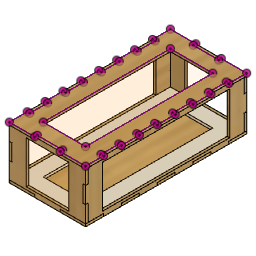
probatio-base-parametric-generator (Autodesk Fusion 360 design; units mm, degrees)
Autodesk Fusion 360 part; units mm, degrees
note: some values were not read from the file. Set by a fixed rule: which sketch regions a step uses.
sketch "Bottom Panel Profile Sketch" plane through (0, 0, 0) normal (0, 0, 1) x (1, 0, 0) in component "Main Box"
  line L0 (0, 0) -> (90, 0)
  line L1 (90, 0) -> (90, 190)
  line L2 (90, 190) -> (0, 190)
  line L3 (0, 190) -> (0, 0)
  dimension "d21" = 90
  dimension "d22" = 190
  constraint horizontal L0
  constraint vertical L1
  constraint horizontal L2
  constraint vertical L3
  constraint coincident L0.start L3.end
  measures "d21" distance of L0.start L0.end
  measures "d22" distance of L0.start L2.end
extrude "Bottom Panel Extrude" add sketch "Bottom Panel Profile Sketch" along normal blind 3 makes body 1 in component "Main Box"
sketch "Bottom Panel Front Fingers Sketch" plane through (0, 0, 0) normal (0, -1, 0) x (1, 0, 0) in component "Main Box"
  line L0 (0, 0) -> (90, 0)
  line L1 (90, 0) -> (90, 3)
  line L2 (90, 3) -> (0, 3)
  line L3 (0, 3) -> (0, 0)
  line L4 (45, 3) -> (45, 0) construction
  line L5 (30, 1.5) -> (60, 1.5) construction
  line L6 (30, 0) -> (60, 0)
  line L7 (60, 0) -> (60, 3)
  line L8 (60, 3) -> (30, 3)
  line L9 (30, 3) -> (30, 0)
  dimension "d25" = 30
  dimension "d26" = 30
  constraint midpoint L2 L4.start
  constraint midpoint L0 L4.end
  constraint perpendicular L4 L5
  constraint midpoint L4 L5
  constraint horizontal L6
  constraint vertical L7
  constraint horizontal L8
  constraint vertical L9
  constraint coincident L2 L7.end
  constraint coincident L0 L6.start
  constraint coincident L5.start L9
  measures "d25" horizontal distance of L7.end L8.end
  measures "d26" horizontal distance of L5.start L5.end
extrude "Bottom Panel Front Finger Extrude" cut sketch "Bottom Panel Front Fingers Sketch" against normal blind 3 contours L0 L2 L6 L7 L8 L9 bodies 1 in component "Main Box"
pattern_linear "Bottom Panel Length Fingers Pattern" count 1 spacing 0 along (1, 0, 0) count 2 spacing 187 along (0, 1, 0) of "Bottom Panel Front Finger Extrude" in component "Main Box"
sketch "Bottom Panel Left Fingers Sketch" plane through (0, 0, 0) normal (-1, 0, 0) x (0, -1, 0) in component "Main Box"
  line L0 (-190, 0) -> (0, 0)
  line L1 (0, 0) -> (0, 3)
  line L2 (0, 3) -> (-190, 3)
  line L3 (-190, 3) -> (-190, 0)
  line L4 (-95, 3) -> (-95, 0) construction
  line L5 (-168.8889, 1.5) -> (-21.1111, 1.5) construction
  line L6 (-21.1111, 0) -> (-42.2222, 0)
  line L7 (-42.2222, 0) -> (-42.2222, 3)
  line L8 (-42.2222, 3) -> (-21.1111, 3)
  line L9 (-21.1111, 3) -> (-21.1111, 0)
  dimension "d33" = 21.1111
  dimension "d34" = 147.7778
  constraint midpoint L2 L4.start
  constraint midpoint L0 L4.end
  constraint perpendicular L4 L5
  constraint midpoint L4 L5
  constraint horizontal L6
  constraint vertical L7
  constraint horizontal L8
  constraint vertical L9
  constraint coincident L2 L7.end
  constraint coincident L0 L6.start
  constraint coincident L5.end L9
  measures "d33" horizontal distance of L6.start L6.end
  measures "d34" horizontal distance of L5.start L5.end
extrude "Bottom Panel Left Finger Extrude" cut sketch "Bottom Panel Left Fingers Sketch" against normal blind 3 contours L0 L2 L6 L7 L8 L9 bodies 1 in component "Main Box"
pattern_linear "Bottom Panel Width Fingers Pattern" count 4 spacing 42.2222 along (0, 1, 0) count 2 spacing 87 along (1, 0, 0) of "Bottom Panel Left Finger Extrude" in component "Main Box"
sketch "Front Panel Profile Sketch" plane through (0, 0, 0) normal (0, 1, 0) x (1, 0, 0) in component "Main Box"
  line L0 (0, 0) -> (90, 0)
  line L1 (90, 0) -> (90, -62)
  line L2 (90, -62) -> (0, -62)
  line L3 (0, -62) -> (0, 0)
  dimension "d41" = 90
  dimension "d42" = 62
  constraint horizontal L0
  constraint vertical L1
  constraint horizontal L2
  constraint vertical L3
  constraint coincident L0.start L3.end
  measures "d41" distance of L0.start L0.end
  measures "d42" distance of L0.start L2.end
extrude "Front Panel Extrude" add sketch "Front Panel Profile Sketch" along normal blind 3 separate body makes body 2 in component "Main Box"
combine "Front Panel Combine" operation cut target body 2 tool bodies 1 keep tools in component "Main Box"
sketch "Front Panel Left Fingers Sketch" plane through (0, 0, 0) normal (0, -1, 0) x (1, 0, 0) in component "Main Box"
  line L0 (90, 3) -> (90, 62)
  line L1 (90, 62) -> (0, 62)
  line L2 (0, 62) -> (0, 3)
  line L3 (0, 3) -> (30, 3)
  line L4 (30, 3) -> (30, 0)
  line L5 (30, 0) -> (60, 0)
  line L6 (60, 0) -> (60, 3)
  line L7 (60, 3) -> (90, 3)
  line L8 (0, 32.5) -> (3, 32.5) construction
  line L9 (1.5, 42.3333) -> (1.5, 22.6667) construction
  line L10 (0, 22.6667) -> (3, 22.6667)
  line L11 (3, 22.6667) -> (3, 42.3333)
  line L12 (3, 42.3333) -> (0, 42.3333)
  line L13 (0, 42.3333) -> (0, 22.6667)
  dimension "d45" = 3
  dimension "d46" = 19.6667
  dimension "d47" = 19.6667
  constraint midpoint L2 L8.start
  constraint perpendicular L2 L8
  constraint perpendicular L8 L9
  constraint midpoint L8 L9
  constraint horizontal L10
  constraint vertical L11
  constraint horizontal L12
  constraint vertical L13
  constraint coincident L2 L10.start
  constraint coincident L9.end L10
  constraint coincident L8.end L11
  measures "d45" distance of L8.start L8.end
  measures "d46" vertical distance of L10.start L12.end
  measures "d47" vertical distance of L9.start L9.end
extrude "Front Panel Left Fingers Extrude" cut sketch "Front Panel Left Fingers Sketch" against normal blind 3 contours L2 L10 L11 L12 L13 bodies 2 in component "Main Box"
pattern_linear "Front Panel Height Fingers Pattern" count 1 spacing 0 along (0, 0, 1) count 2 spacing 87 along (1, 0, 0) of "Front Panel Left Fingers Extrude" in component "Main Box"
pattern_linear "Front Panel Pattern" count 2 spacing 187 along (0, 1, 0) of bodies 2 makes body 3 in component "Main Box"
sketch "Left Panel Profile Sketch" plane through (0, 0, 0) normal (1, 0, 0) x (0, 1, 0) in component "Main Box"
  line L0 (0, 0) -> (190, 0)
  line L1 (190, 0) -> (190, 62)
  line L2 (190, 62) -> (0, 62)
  line L3 (0, 62) -> (0, 0)
  dimension "d58" = 190
  dimension "d59" = 62
  constraint horizontal L0
  constraint vertical L1
  constraint horizontal L2
  constraint vertical L3
  constraint coincident L0.start L3.end
  measures "d58" distance of L0.start L0.end
  measures "d59" distance of L0.start L2.end
extrude "Left Panel Extrude" add sketch "Left Panel Profile Sketch" along normal blind 3 separate body makes body 4 in component "Main Box"
sketch "Left Panel Front Fingers Sketch" plane through (0, 0, 0) normal (0, -1, 0) x (1, 0, 0) in component "Main Box"
  line L0 (0, 62) -> (0, 0)
  line L1 (0, 0) -> (3, 0)
  line L2 (3, 0) -> (3, 62)
  line L3 (3, 62) -> (0, 62)
  line L4 (0, 62) -> (3, 62)
  line L5 (3, 62) -> (3, 42.3333)
  line L6 (3, 42.3333) -> (0, 42.3333)
  line L7 (0, 42.3333) -> (0, 62)
  dimension "d72" = 19.6667
  constraint horizontal L4
  constraint vertical L5
  constraint horizontal L6
  constraint vertical L7
  constraint coincident L2 L5.end
  constraint coincident L0.start L3.end
  measures "d72" vertical distance of L0.start L6.end
extrude "Left Panel Front Fingers Extrude" cut sketch "Left Panel Front Fingers Sketch" against normal blind 3 contours L0 L2 L3 L4 L5 L6 L7 bodies 4 in component "Main Box"
pattern_linear "Left Panel Slots Pattern" count 2 spacing 187 along (0, 1, 0) of "Left Panel Front Fingers Extrude" in component "Main Box"
combine "Left Panel Combine" operation cut target body 4 tool bodies 3 1 2 keep tools in component "Main Box"
extrude "Extrude11" add 1 faces at (0, 91.4815, 42.3333) along direction (-1, 0, 0) blind 3 from surface at -90 separate body on bodies 4 makes body 5 in component "Main Box"
extrude "Extrude9" cut 1 faces at (50, 29.1481, 3) along direction (0, 0, -1) blind 3 from surface at -59 on bodies 1 bodies 2 3 4 5 in component "Main Box"
extrude "Extrude12" add 1 faces at (50, 29.1481, 0) along direction (0, 0, -1) blind 3 from surface at -62 separate body on bodies 1 makes body 6 in component "Main Box"
sketch "Sketch8" plane through (0, 190, 0) normal (0, 1, 0) x (-1, 0, 0) in component "Main Box"
  line L0 (-90, 59) -> (-90, 42.3333)
  line L1 (-90, 42.3333) -> (-87, 42.3333)
  line L2 (-87, 42.3333) -> (-87, 22.6667)
  line L3 (-87, 22.6667) -> (-90, 22.6667)
  line L4 (-90, 22.6667) -> (-90, 3)
  line L5 (-90, 3) -> (-60, 3)
  line L6 (-60, 3) -> (-60, 0)
  line L7 (-60, 0) -> (-30, 0)
  line L8 (-30, 0) -> (-30, 3)
  line L9 (-30, 3) -> (0, 3)
  line L10 (0, 3) -> (0, 22.6667)
  line L11 (0, 22.6667) -> (-3, 22.6667)
  line L12 (-3, 22.6667) -> (-3, 42.3333)
  line L13 (-3, 42.3333) -> (0, 42.3333)
  line L14 (0, 42.3333) -> (0, 59)
  line L15 (-30, 62) -> (-60, 62)
  line L16 (-90, 59) -> (0, 3) construction
  line L17 (0, 59) -> (-90, 3) construction
  line L18 (-20, 56) -> (-70, 56)
  line L19 (-70, 56) -> (-70, 6)
  line L20 (-70, 6) -> (-20, 6)
  line L21 (-20, 6) -> (-20, 56)
  line L22 (-20, 56) -> (-70, 6) construction
  line L23 (-70, 56) -> (-20, 6) construction
  line L24 (0, 59) -> (-30, 59)
  line L25 (-30, 59) -> (-30, 62)
  line L26 (-60, 62) -> (-60, 59)
  line L27 (-60, 59) -> (-90, 59)
  point P0 (-45, 31)
  dimension "d118" = 50
  dimension "d119" = 50
  constraint coincident L0.start L16.start
  constraint coincident L9.end L10.start
  constraint coincident L14.end L17.start
  constraint coincident L4.end L5.start
  constraint perpendicular L18 L19
  constraint parallel L18 L20
  constraint parallel L19 L21
  constraint horizontal L18
  constraint coincident L22 P0
  constraint coincident L23 P0
  constraint midpoint L16 P0
  measures "d118" distance of L18.end L19.end
  measures "d119" distance of L19.end L20.end
extrude "Extrude10" cut sketch "Sketch8" against normal blind 3 contours L18 L19 L20 L21 bodies 3 in component "Main Box"
sketch "Sketch9" plane through (0, 0, 62) normal (0, 0, 1) x (-1, 0, 0) in component "Main Box"
  line L0 (-90, -190) -> (-60, -190)
  line L1 (-60, -190) -> (-60, -187)
  line L2 (-60, -187) -> (-30, -187)
  line L3 (-30, -187) -> (-30, -190)
  line L4 (-30, -190) -> (0, -190)
  line L5 (0, -63.3333) -> (0, -42.2222)
  line L6 (0, -42.2222) -> (-3, -42.2222)
  line L7 (-3, -42.2222) -> (-3, -21.1111)
  line L8 (-3, -21.1111) -> (0, -21.1111)
  line L9 (0, -21.1111) -> (0, 0)
  line L10 (0, 0) -> (-30, 0)
  line L11 (-30, 0) -> (-30, -3)
  line L12 (-30, -3) -> (-60, -3)
  line L13 (-60, -3) -> (-60, 0)
  line L14 (-60, 0) -> (-90, 0)
  line L15 (-90, 0) -> (-90, -21.1111)
  line L16 (-90, -21.1111) -> (-87, -21.1111)
  line L17 (-87, -21.1111) -> (-87, -42.2222)
  line L18 (-87, -42.2222) -> (-90, -42.2222)
  line L19 (-90, -42.2222) -> (-90, -63.3333)
  line L20 (-90, -147.7778) -> (-87, -147.7778)
  line L21 (-87, -147.7778) -> (-87, -168.8889)
  line L22 (-87, -168.8889) -> (-90, -168.8889)
  line L23 (-90, -168.8889) -> (-90, -190)
  line L24 (0, -190) -> (0, -168.8889)
  line L25 (0, -168.8889) -> (-3, -168.8889)
  line L26 (-3, -168.8889) -> (-3, -147.7778)
  line L27 (-3, -147.7778) -> (0, -147.7778)
  line L28 (0, -147.7778) -> (0, -126.6667)
  line L29 (0, -126.6667) -> (-3, -126.6667)
  line L30 (-3, -126.6667) -> (-3, -105.5556)
  line L31 (-3, -105.5556) -> (0, -105.5556)
  line L32 (0, -105.5556) -> (0, -84.4444)
  line L33 (0, -84.4444) -> (-3, -84.4444)
  line L34 (-3, -84.4444) -> (-3, -63.3333)
  line L35 (-3, -63.3333) -> (0, -63.3333)
  line L36 (-90, -63.3333) -> (-87, -63.3333)
  line L37 (-87, -63.3333) -> (-87, -84.4444)
  line L38 (-87, -84.4444) -> (-90, -84.4444)
  line L39 (-90, -84.4444) -> (-90, -105.5556)
  line L40 (-90, -105.5556) -> (-87, -105.5556)
  line L41 (-87, -105.5556) -> (-87, -126.6667)
  line L42 (-87, -126.6667) -> (-90, -126.6667)
  line L43 (-90, -126.6667) -> (-90, -147.7778)
  line L44 (0, -190) -> (-90, 0) construction
  line L45 (-70, -20) -> (-20, -20)
  line L46 (-20, -20) -> (-20, -170)
  line L47 (-20, -170) -> (-70, -170)
  line L48 (-70, -170) -> (-70, -20)
  line L49 (-70, -20) -> (-20, -170) construction
  line L50 (-20, -20) -> (-70, -170) construction
  point P0 (-45, -95)
  dimension "d152" = 50
  dimension "d153" = 150
  constraint coincident L4.end L24.start
  constraint coincident L14.end L15.start
  constraint perpendicular L45 L46
  constraint parallel L45 L47
  constraint parallel L46 L48
  constraint horizontal L45
  constraint coincident L49 P0
  constraint coincident L50 P0
  constraint midpoint L44 P0
  measures "d152" distance of L46.end L47.end
  measures "d153" distance of L45.end L46.end
extrude "Extrude13" cut sketch "Sketch9" against normal blind 3 contours L45 L46 L47 L48 bodies 6 in component "Main Box"
sketch "Sketch10" plane through (0, 0, 0) normal (0, -1, 0) x (1, 0, 0) in component "Main Box"
  line L0 (30, 59) -> (0, 59)
  line L1 (0, 59) -> (0, 42.3333)
  line L2 (0, 42.3333) -> (3, 42.3333)
  line L3 (3, 42.3333) -> (3, 22.6667)
  line L4 (3, 22.6667) -> (0, 22.6667)
  line L5 (0, 22.6667) -> (0, 3)
  line L6 (0, 3) -> (30, 3)
  line L7 (30, 3) -> (30, 0)
  line L8 (30, 0) -> (60, 0)
  line L9 (60, 0) -> (60, 3)
  line L10 (60, 3) -> (90, 3)
  line L11 (90, 3) -> (90, 22.6667)
  line L12 (90, 22.6667) -> (87, 22.6667)
  line L13 (87, 22.6667) -> (87, 42.3333)
  line L14 (87, 42.3333) -> (90, 42.3333)
  line L15 (90, 42.3333) -> (90, 59)
  line L16 (90, 59) -> (60, 59)
  line L17 (60, 59) -> (60, 62)
  line L18 (60, 62) -> (30, 62)
  line L19 (30, 62) -> (30, 59)
  line L20 (90, 59) -> (0, 3) construction
  line L21 (70, 6) -> (20, 6)
  line L22 (20, 6) -> (20, 56)
  line L23 (20, 56) -> (70, 56)
  line L24 (70, 56) -> (70, 6)
  line L25 (70, 6) -> (20, 56) construction
  line L26 (20, 6) -> (70, 56) construction
  point P0 (45, 31)
  dimension "d150" = 50
  dimension "d151" = 50
  constraint coincident L15.end L16.start
  constraint coincident L5.end L6.start
  constraint perpendicular L21 L22
  constraint parallel L21 L23
  constraint parallel L22 L24
  constraint horizontal L21
  constraint coincident L25 P0
  constraint coincident L26 P0
  constraint midpoint L20 P0
  measures "d150" distance of L22.end L23.end
  measures "d151" distance of L21.end L22.end
extrude "Extrude14" cut sketch "Sketch10" against normal blind 3 contours L21 L22 L23 L24 bodies 2 in component "Main Box"
sketch "Sketch11" plane through (90, 0, 0) normal (1, 0, 0) x (0, 1, 0) in component "Main Box"
  line L0 (187, 59) -> (168.8889, 59)
  line L1 (42.2222, 59) -> (42.2222, 62)
  line L2 (42.2222, 62) -> (21.1111, 62)
  line L3 (21.1111, 62) -> (21.1111, 59)
  line L4 (21.1111, 59) -> (3, 59)
  line L5 (3, 59) -> (3, 42.3333)
  line L6 (3, 42.3333) -> (0, 42.3333)
  line L7 (0, 42.3333) -> (0, 22.6667)
  line L8 (0, 22.6667) -> (3, 22.6667)
  line L9 (3, 22.6667) -> (3, 3)
  line L10 (3, 3) -> (21.1111, 3)
  line L11 (21.1111, 3) -> (21.1111, 0)
  line L12 (21.1111, 0) -> (42.2222, 0)
  line L13 (42.2222, 0) -> (42.2222, 3)
  line L14 (126.6667, 3) -> (147.7778, 3)
  line L15 (187, 3) -> (187, 22.6667)
  line L16 (187, 22.6667) -> (190, 22.6667)
  line L17 (190, 22.6667) -> (190, 42.3333)
  line L18 (190, 42.3333) -> (187, 42.3333)
  line L19 (187, 42.3333) -> (187, 59)
  line L20 (3, 59) -> (147.7778, 3) construction
  line L21 (187, 59) -> (3, 3) construction
  line L22 (170, 56) -> (20, 56)
  line L23 (20, 56) -> (20, 6)
  line L24 (20, 6) -> (170, 6)
  line L25 (170, 6) -> (170, 56)
  line L26 (170, 56) -> (20, 6) construction
  line L27 (20, 56) -> (170, 6) construction
  line L28 (168.8889, 59) -> (168.8889, 62)
  line L29 (147.7778, 62) -> (147.7778, 59)
  line L30 (147.7778, 59) -> (126.6667, 59)
  line L31 (126.6667, 59) -> (126.6667, 62)
  line L32 (126.6667, 62) -> (105.5556, 62)
  line L33 (105.5556, 62) -> (105.5556, 59)
  line L34 (105.5556, 59) -> (84.4444, 59)
  line L35 (84.4444, 59) -> (84.4444, 62)
  line L36 (84.4444, 62) -> (63.3333, 62)
  line L37 (63.3333, 62) -> (63.3333, 59)
  line L38 (63.3333, 59) -> (42.2222, 59)
  line L39 (42.2222, 3) -> (63.3333, 3)
  line L40 (63.3333, 3) -> (63.3333, 0)
  line L41 (63.3333, 0) -> (84.4444, 0)
  line L42 (84.4444, 0) -> (84.4444, 3)
  line L43 (84.4444, 3) -> (105.5556, 3)
  line L44 (105.5556, 3) -> (105.5556, 0)
  line L45 (105.5556, 0) -> (126.6667, 0)
  line L46 (126.6667, 0) -> (126.6667, 3)
  line L47 (147.7778, 3) -> (147.7778, 0)
  line L48 (147.7778, 0) -> (168.8889, 0)
  line L49 (168.8889, 0) -> (168.8889, 3)
  line L50 (168.8889, 62) -> (147.7778, 62)
  line L51 (168.8889, 3) -> (187, 3)
  point P0 (95, 31)
  dimension "d136" = 150
  dimension "d137" = 50
  constraint coincident L4.end L5.start
  constraint coincident L14.end L20.end
  constraint coincident L0.start L19.end
  constraint coincident L9.end L10.start
  constraint perpendicular L22 L23
  constraint parallel L22 L24
  constraint parallel L23 L25
  constraint horizontal L22
  constraint coincident L26 P0
  constraint coincident L27 P0
  constraint midpoint L21 P0
  measures "d136" distance of L23.end L24.end
  measures "d137" distance of L22.end L23.end
extrude "Extrude15" cut sketch "Sketch11" against normal blind 3 contours L22 L23 L24 L25 bodies 5 in component "Main Box"
sketch "Sketch12" plane through (0, 0, 0) normal (-1, 0, 0) x (0, -1, 0) in component "Main Box"
  line L0 (-187, 59) -> (-187, 42.3333)
  line L1 (-187, 42.3333) -> (-190, 42.3333)
  line L2 (-190, 42.3333) -> (-190, 22.6667)
  line L3 (-190, 22.6667) -> (-187, 22.6667)
  line L4 (-187, 22.6667) -> (-187, 3)
  line L5 (-187, 3) -> (-168.8889, 3)
  line L6 (-42.2222, 3) -> (-42.2222, 0)
  line L7 (-42.2222, 0) -> (-21.1111, 0)
  line L8 (-21.1111, 0) -> (-21.1111, 3)
  line L9 (-21.1111, 3) -> (-3, 3)
  line L10 (-3, 3) -> (-3, 22.6667)
  line L11 (-3, 22.6667) -> (0, 22.6667)
  line L12 (0, 22.6667) -> (0, 42.3333)
  line L13 (0, 42.3333) -> (-3, 42.3333)
  line L14 (-3, 42.3333) -> (-3, 59)
  line L15 (-21.1111, 59) -> (-21.1111, 62)
  line L16 (-21.1111, 62) -> (-42.2222, 62)
  line L17 (-42.2222, 62) -> (-42.2222, 59)
  line L18 (-42.2222, 59) -> (-63.3333, 59)
  line L19 (-187, 59) -> (-3, 3) construction
  line L20 (-136.5807, 56.5348) -> (-187, 3) construction
  line L21 (-20, 56) -> (-170, 56)
  line L22 (-170, 56) -> (-170, 6)
  line L23 (-170, 6) -> (-20, 6)
  line L24 (-20, 6) -> (-20, 56)
  line L25 (-20, 56) -> (-170, 6) construction
  line L26 (-170, 56) -> (-20, 6) construction
  line L27 (-3, 59) -> (-21.1111, 59)
  line L28 (-168.8889, 3) -> (-168.8889, 0)
  line L29 (-147.7778, 0) -> (-147.7778, 3)
  line L30 (-147.7778, 3) -> (-126.6667, 3)
  line L31 (-126.6667, 3) -> (-126.6667, 0)
  line L32 (-126.6667, 0) -> (-105.5556, 0)
  line L33 (-105.5556, 0) -> (-105.5556, 3)
  line L34 (-105.5556, 3) -> (-84.4444, 3)
  line L35 (-84.4444, 3) -> (-84.4444, 0)
  line L36 (-84.4444, 0) -> (-63.3333, 0)
  line L37 (-63.3333, 0) -> (-63.3333, 3)
  line L38 (-63.3333, 3) -> (-42.2222, 3)
  line L39 (-63.3333, 59) -> (-63.3333, 62)
  line L40 (-63.3333, 62) -> (-84.4444, 62)
  line L41 (-84.4444, 62) -> (-84.4444, 59)
  line L42 (-84.4444, 59) -> (-105.5556, 59)
  line L43 (-105.5556, 59) -> (-105.5556, 62)
  line L44 (-105.5556, 62) -> (-126.6667, 62)
  line L45 (-126.6667, 62) -> (-126.6667, 59)
  line L46 (-126.6667, 59) -> (-147.7778, 59)
  line L47 (-147.7778, 59) -> (-147.7778, 62)
  line L48 (-147.7778, 62) -> (-168.8889, 62)
  line L49 (-168.8889, 62) -> (-168.8889, 59)
  line L50 (-168.8889, 0) -> (-147.7778, 0)
  line L51 (-168.8889, 59) -> (-187, 59)
  point P0 (-95, 31)
  dimension "d140" = 150
  dimension "d141" = 50
  constraint coincident L0.start L19.start
  constraint coincident L9.end L10.start
  constraint coincident L4.end L5.start
  constraint perpendicular L21 L22
  constraint parallel L21 L23
  constraint parallel L22 L24
  constraint horizontal L21
  constraint coincident L25 P0
  constraint coincident L26 P0
  constraint midpoint L19 P0
  measures "d140" distance of L22.end L23.end
  measures "d141" distance of L21.end L22.end
extrude "Extrude16" cut sketch "Sketch12" against normal blind 3 contours L21 L22 L23 L24 bodies 4 in component "Main Box"
sketch "Sketch13" plane through (0, 0, 3) normal (0, 0, 1) x (-1, 0, 0) in component "Main Box"
  line L0 (-90, -190) -> (-60, -190)
  line L1 (-60, -190) -> (-60, -187)
  line L2 (-60, -187) -> (-30, -187)
  line L3 (-30, -187) -> (-30, -190)
  line L4 (-30, -190) -> (0, -190)
  line L5 (0, -190) -> (0, -168.8889)
  line L6 (0, -42.2222) -> (-3, -42.2222)
  line L7 (-3, -42.2222) -> (-3, -21.1111)
  line L8 (-3, -21.1111) -> (0, -21.1111)
  line L9 (0, -21.1111) -> (0, 0)
  line L10 (0, 0) -> (-30, 0)
  line L11 (-30, 0) -> (-30, -3)
  line L12 (-30, -3) -> (-60, -3)
  line L13 (-60, -3) -> (-60, 0)
  line L14 (-60, 0) -> (-90, 0)
  line L15 (-90, 0) -> (-90, -21.1111)
  line L16 (-90, -21.1111) -> (-87, -21.1111)
  line L17 (-87, -21.1111) -> (-87, -42.2222)
  line L18 (-87, -42.2222) -> (-90, -42.2222)
  line L19 (-90, -42.2222) -> (-90, -63.3333)
  line L20 (0, -190) -> (-90, 0) construction
  line L21 (-90, -190) -> (0, 0) construction
  line L22 (-87, -3) -> (-3, -3)
  line L23 (-3, -3) -> (-3, -187)
  line L24 (-3, -187) -> (-87, -187)
  line L25 (-87, -187) -> (-87, -3)
  line L26 (-87, -3) -> (-3, -187) construction
  line L27 (-3, -3) -> (-87, -187) construction
  line L28 (-70, -20) -> (-20, -20)
  line L29 (-20, -20) -> (-20, -170)
  line L30 (-20, -170) -> (-70, -170)
  line L31 (-70, -170) -> (-70, -20)
  line L32 (-70, -20) -> (-20, -170) construction
  line L33 (-20, -20) -> (-70, -170) construction
  line L34 (-90, -147.7778) -> (-87, -147.7778)
  line L35 (-87, -147.7778) -> (-87, -168.8889)
  line L36 (-87, -168.8889) -> (-90, -168.8889)
  line L37 (0, -168.8889) -> (-3, -168.8889)
  line L38 (-3, -168.8889) -> (-3, -147.7778)
  line L39 (-3, -147.7778) -> (0, -147.7778)
  line L40 (0, -147.7778) -> (0, -126.6667)
  line L41 (0, -126.6667) -> (-3, -126.6667)
  line L42 (-3, -126.6667) -> (-3, -105.5556)
  line L43 (-3, -105.5556) -> (0, -105.5556)
  line L44 (0, -105.5556) -> (0, -84.4444)
  line L45 (0, -84.4444) -> (-3, -84.4444)
  line L46 (-3, -84.4444) -> (-3, -63.3333)
  line L47 (-3, -63.3333) -> (0, -63.3333)
  line L48 (0, -63.3333) -> (0, -42.2222)
  line L49 (-90, -63.3333) -> (-87, -63.3333)
  line L50 (-87, -63.3333) -> (-87, -84.4444)
  line L51 (-87, -84.4444) -> (-90, -84.4444)
  line L52 (-90, -84.4444) -> (-90, -105.5556)
  line L53 (-90, -105.5556) -> (-87, -105.5556)
  line L54 (-87, -105.5556) -> (-87, -126.6667)
  line L55 (-87, -126.6667) -> (-90, -126.6667)
  line L56 (-90, -126.6667) -> (-90, -147.7778)
  line L57 (-90, -168.8889) -> (-90, -190)
  point P0 (-45, -95)
  point P1 (-45, -95)
  dimension "d144" = 84
  dimension "d145" = 184
  dimension "d146" = 50
  dimension "d147" = 150
  constraint coincident L4.end L5.start
  constraint coincident L14.end L15.start
  constraint coincident L0.start L21.start
  constraint coincident L9.end L10.start
  constraint perpendicular L22 L23
  constraint parallel L22 L24
  constraint parallel L23 L25
  constraint horizontal L22
  constraint coincident L26 P1
  constraint coincident L27 P1
  constraint midpoint L21 P1
  constraint perpendicular L28 L29
  constraint parallel L28 L30
  constraint parallel L29 L31
  constraint horizontal L28
  constraint coincident L32 P1
  constraint coincident L33 P1
  constraint coincident P1 P0
  measures "d144" distance of L23.end L24.end
  measures "d145" distance of L22.end L23.end
  measures "d146" distance of L29.end L30.end
  measures "d147" distance of L28.end L29.end
extrude "Extrude17" add sketch "Sketch13" along normal blind 3 separate body contours L2 L7 L12 L17 L22 L23 L24 L25 L35 L38 L42 L46 L50 L54 makes body 7 in component "Main Box"
sketch "Top Profile" plane through (0, 0, 62) normal (0, 0, 1) x (-1, 0, 0)
  line L0 (-20, -20) -> (-20, -170)
  line L1 (-20, -170) -> (-70, -170)
  line L2 (-70, -170) -> (-70, -20)
  line L3 (-70, -20) -> (-20, -20)
  line L4 (-90, -147.7778) -> (-87, -147.7778)
  line L5 (-87, -147.7778) -> (-87, -168.8889)
  line L6 (-87, -168.8889) -> (-90, -168.8889)
  line L7 (-90, -168.8889) -> (-90, -190)
  line L8 (-90, -190) -> (-60, -190)
  line L9 (-60, -190) -> (-60, -187)
  line L10 (-60, -187) -> (-30, -187)
  line L11 (-30, -187) -> (-30, -190)
  line L12 (-30, -190) -> (0, -190)
  line L13 (0, -190) -> (0, -168.8889)
  line L14 (0, -168.8889) -> (-3, -168.8889)
  line L15 (-3, -168.8889) -> (-3, -147.7778)
  line L16 (-3, -147.7778) -> (0, -147.7778)
  line L17 (0, -147.7778) -> (0, -126.6667)
  line L18 (0, -126.6667) -> (-3, -126.6667)
  line L19 (-3, -126.6667) -> (-3, -105.5556)
  line L20 (-3, -105.5556) -> (0, -105.5556)
  line L21 (0, -105.5556) -> (0, -84.4444)
  line L22 (0, -84.4444) -> (-3, -84.4444)
  line L23 (-3, -84.4444) -> (-3, -63.3333)
  line L24 (-3, -63.3333) -> (0, -63.3333)
  line L25 (0, -63.3333) -> (0, -42.2222)
  line L26 (0, -42.2222) -> (-3, -42.2222)
  line L27 (-3, -42.2222) -> (-3, -21.1111)
  line L28 (-3, -21.1111) -> (0, -21.1111)
  line L29 (0, -21.1111) -> (0, 0)
  line L30 (0, 0) -> (-30, 0)
  line L31 (-30, 0) -> (-30, -3)
  line L32 (-30, -3) -> (-60, -3)
  line L33 (-60, -3) -> (-60, 0)
  line L34 (-60, 0) -> (-90, 0)
  line L35 (-90, 0) -> (-90, -21.1111)
  line L36 (-90, -21.1111) -> (-87, -21.1111)
  line L37 (-87, -21.1111) -> (-87, -42.2222)
  line L38 (-87, -42.2222) -> (-90, -42.2222)
  line L39 (-90, -42.2222) -> (-90, -63.3333)
  line L40 (-90, -63.3333) -> (-87, -63.3333)
  line L41 (-87, -63.3333) -> (-87, -84.4444)
  line L42 (-87, -84.4444) -> (-90, -84.4444)
  line L43 (-90, -84.4444) -> (-90, -105.5556)
  line L44 (-90, -105.5556) -> (-87, -105.5556)
  line L45 (-87, -105.5556) -> (-87, -126.6667)
  line L46 (-87, -126.6667) -> (-90, -126.6667)
  line L47 (-90, -126.6667) -> (-90, -147.7778)
sketch "Side A Profile" plane through (0, 0, 0) normal (-1, 0, 0) x (0, -1, 0)
  line L0 (-170, 56) -> (-20, 56)
  line L1 (-20, 56) -> (-20, 6)
  line L2 (-20, 6) -> (-170, 6)
  line L3 (-170, 6) -> (-170, 56)
  line L4 (-168.8889, 59) -> (-187, 59)
  line L5 (-187, 59) -> (-187, 42.3333)
  line L6 (-187, 42.3333) -> (-190, 42.3333)
  line L7 (-190, 42.3333) -> (-190, 22.6667)
  line L8 (-190, 22.6667) -> (-187, 22.6667)
  line L9 (-187, 22.6667) -> (-187, 3)
  line L10 (-187, 3) -> (-168.8889, 3)
  line L11 (-168.8889, 3) -> (-168.8889, 0)
  line L12 (-168.8889, 0) -> (-147.7778, 0)
  line L13 (-147.7778, 0) -> (-147.7778, 3)
  line L14 (-147.7778, 3) -> (-126.6667, 3)
  line L15 (-126.6667, 3) -> (-126.6667, 0)
  line L16 (-126.6667, 0) -> (-105.5556, 0)
  line L17 (-105.5556, 0) -> (-105.5556, 3)
  line L18 (-105.5556, 3) -> (-84.4444, 3)
  line L19 (-84.4444, 3) -> (-84.4444, 0)
  line L20 (-84.4444, 0) -> (-63.3333, 0)
  line L21 (-63.3333, 0) -> (-63.3333, 3)
  line L22 (-63.3333, 3) -> (-42.2222, 3)
  line L23 (-42.2222, 3) -> (-42.2222, 0)
  line L24 (-42.2222, 0) -> (-21.1111, 0)
  line L25 (-21.1111, 0) -> (-21.1111, 3)
  line L26 (-21.1111, 3) -> (-3, 3)
  line L27 (-3, 3) -> (-3, 22.6667)
  line L28 (-3, 22.6667) -> (0, 22.6667)
  line L29 (0, 22.6667) -> (0, 42.3333)
  line L30 (0, 42.3333) -> (-3, 42.3333)
  line L31 (-3, 42.3333) -> (-3, 59)
  line L32 (-3, 59) -> (-21.1111, 59)
  line L33 (-21.1111, 59) -> (-21.1111, 62)
  line L34 (-21.1111, 62) -> (-42.2222, 62)
  line L35 (-42.2222, 62) -> (-42.2222, 59)
  line L36 (-42.2222, 59) -> (-63.3333, 59)
  line L37 (-63.3333, 59) -> (-63.3333, 62)
  line L38 (-63.3333, 62) -> (-84.4444, 62)
  line L39 (-84.4444, 62) -> (-84.4444, 59)
  line L40 (-84.4444, 59) -> (-105.5556, 59)
  line L41 (-105.5556, 59) -> (-105.5556, 62)
  line L42 (-105.5556, 62) -> (-126.6667, 62)
  line L43 (-126.6667, 62) -> (-126.6667, 59)
  line L44 (-126.6667, 59) -> (-147.7778, 59)
  line L45 (-147.7778, 59) -> (-147.7778, 62)
  line L46 (-147.7778, 62) -> (-168.8889, 62)
  line L47 (-168.8889, 62) -> (-168.8889, 59)
sketch "Side B Profile" plane through (0, 0, 0) normal (0, -1, 0) x (1, 0, 0)
  line L0 (20, 6) -> (20, 56)
  line L1 (20, 56) -> (70, 56)
  line L2 (70, 56) -> (70, 6)
  line L3 (70, 6) -> (20, 6)
  line L4 (30, 59) -> (0, 59)
  line L5 (0, 59) -> (0, 42.3333)
  line L6 (0, 42.3333) -> (3, 42.3333)
  line L7 (3, 42.3333) -> (3, 22.6667)
  line L8 (3, 22.6667) -> (0, 22.6667)
  line L9 (0, 22.6667) -> (0, 3)
  line L10 (0, 3) -> (30, 3)
  line L11 (30, 3) -> (30, 0)
  line L12 (30, 0) -> (60, 0)
  line L13 (60, 0) -> (60, 3)
  line L14 (60, 3) -> (90, 3)
  line L15 (90, 3) -> (90, 22.6667)
  line L16 (90, 22.6667) -> (87, 22.6667)
  line L17 (87, 22.6667) -> (87, 42.3333)
  line L18 (87, 42.3333) -> (90, 42.3333)
  line L19 (90, 42.3333) -> (90, 59)
  line L20 (90, 59) -> (60, 59)
  line L21 (60, 59) -> (60, 62)
  line L22 (60, 62) -> (30, 62)
  line L23 (30, 62) -> (30, 59)
sketch "Bottom Profile" plane through (0, 0, 0) normal (0, 0, -1) x (1, 0, 0)
  line L0 (87, -147.7778) -> (90, -147.7778)
  line L1 (90, -147.7778) -> (90, -126.6667)
  line L2 (90, -126.6667) -> (87, -126.6667)
  line L3 (87, -126.6667) -> (87, -105.5556)
  line L4 (87, -105.5556) -> (90, -105.5556)
  line L5 (90, -105.5556) -> (90, -84.4444)
  line L6 (90, -84.4444) -> (87, -84.4444)
  line L7 (87, -84.4444) -> (87, -63.3333)
  line L8 (87, -63.3333) -> (90, -63.3333)
  line L9 (90, -63.3333) -> (90, -42.2222)
  line L10 (90, -42.2222) -> (87, -42.2222)
  line L11 (87, -42.2222) -> (87, -21.1111)
  line L12 (87, -21.1111) -> (90, -21.1111)
  line L13 (90, -21.1111) -> (90, 0)
  line L14 (90, 0) -> (60, 0)
  line L15 (60, 0) -> (60, -3)
  line L16 (60, -3) -> (30, -3)
  line L17 (30, -3) -> (30, 0)
  line L18 (30, 0) -> (0, 0)
  line L19 (0, 0) -> (0, -21.1111)
  line L20 (0, -21.1111) -> (3, -21.1111)
  line L21 (3, -21.1111) -> (3, -42.2222)
  line L22 (3, -42.2222) -> (0, -42.2222)
  line L23 (0, -42.2222) -> (0, -63.3333)
  line L24 (0, -63.3333) -> (3, -63.3333)
  line L25 (3, -63.3333) -> (3, -84.4444)
  line L26 (3, -84.4444) -> (0, -84.4444)
  line L27 (0, -84.4444) -> (0, -105.5556)
  line L28 (0, -105.5556) -> (3, -105.5556)
  line L29 (3, -105.5556) -> (3, -126.6667)
  line L30 (3, -126.6667) -> (0, -126.6667)
  line L31 (0, -126.6667) -> (0, -147.7778)
  line L32 (0, -147.7778) -> (3, -147.7778)
  line L33 (3, -147.7778) -> (3, -168.8889)
  line L34 (3, -168.8889) -> (0, -168.8889)
  line L35 (0, -168.8889) -> (0, -190)
  line L36 (0, -190) -> (30, -190)
  line L37 (30, -190) -> (30, -187)
  line L38 (30, -187) -> (60, -187)
  line L39 (60, -187) -> (60, -190)
  line L40 (60, -190) -> (90, -190)
  line L41 (90, -190) -> (90, -168.8889)
  line L42 (90, -168.8889) -> (87, -168.8889)
  line L43 (87, -168.8889) -> (87, -147.7778)
sketch "Internal Margin Profile" plane through (0, 0, 6) normal (0, 0, 1) x (-1, 0, 0)
  line L0 (-20, -170) -> (-70, -170)
  line L1 (-70, -170) -> (-70, -20)
  line L2 (-70, -20) -> (-20, -20)
  line L3 (-20, -20) -> (-20, -170)
  line L4 (-87, -187) -> (-3, -187)
  line L5 (-3, -187) -> (-3, -3)
  line L6 (-3, -3) -> (-87, -3)
  line L7 (-87, -3) -> (-87, -187)
component "Main Box" placed x (1, 0, 0) y (0, 1, 0) z (0, 0, 1) at (0, 0, 0)
equation "length = outerLength" comment "User defined length of the box"
equation "width = outerWidth" comment "User defined width of the box"
equation "height = outerHeight" comment "User defined height of the box"
equation "thickness = 3.0 mm" comment "User defined thickness of the outer box material"
equation "ciheight = height - thickness" comment "Calculated inner height of the box"
equation "ciwidth = width - thickness * 2" comment "Calculated inner width of the box"
equation "cilength = length - thickness * 2" comment "Calculated inner length of the box"
equation "fingerw = thickness * 6" comment "Optimal finger width"
equation "lfingers = max(3; ( floor(ceil(length / fingerw) / 2) * 2 ) - 1)" comment "Length axis: number of fingers"
equation "lfingerw = length / lfingers" comment "Length axis: actual finger width"
equation "lnotches = floor(lfingers / 2)" comment "Length axis: number of notches along the edge"
equation "lnotchl = ( lfingers - 2 ) * lfingerw" comment "Length axis: length of the notch reference line"
equation "wfingers = max(3; ( floor(ceil(width / fingerw) / 2) * 2 ) - 1)" comment "Width axis: number of fingers"
equation "wfingerw = width / wfingers" comment "Width axis: actual finger width"
equation "wnotches = floor(wfingers / 2)" comment "Width axis: number of notches along the edge"
equation "wnotchl = ( wfingers - 2 ) * wfingerw" comment "Width axis: length of the notch reference line"
equation "hfingers = max(3; ( floor(ceil(ciheight / fingerw) / 2) * 2 ) - 1)" comment "Height axis: number of fingers"
equation "hfingerw = ciheight / hfingers" comment "Height axis: actual finger width"
equation "hnotches = floor(hfingers / 2)" comment "Height axis: number of notches along the edge"
equation "hnotchl = ( hfingers - 2 ) * hfingerw" comment "Height axis: length of the notch reference line"
equation "d21 = length"
equation "d22 = width"
equation "d23 = thickness"
equation "d25 = lfingerw"
equation "d26 = lnotchl"
equation "d27 = -thickness"
equation "d29 = lnotches"
equation "d31 = lnotchl - lfingerw"
equation "d32 = width - thickness"
equation "d33 = wfingerw"
equation "d34 = wnotchl"
equation "d35 = -thickness"
equation "d37 = wnotches"
equation "d38 = 2 + cldividers"
equation "d39 = wnotchl - wfingerw"
equation "d40 = -( length - thickness )"
equation "d41 = length"
equation "d42 = height"
equation "d43 = thickness"
equation "d45 = thickness"
equation "d46 = hfingerw"
equation "d47 = hnotchl"
equation "d48 = -thickness"
equation "d50 = hnotches"
equation "d51 = 2 + cldividers"
equation "d52 = hnotchl - hfingerw"
equation "d53 = length - thickness"
equation "d56 = width - thickness"
equation "d58 = width"
equation "d59 = height"
equation "d60 = thickness"
equation "lcompartments = ldividers + 1" comment "Length axis: Number of compartments"
equation "clcompartments = max(0; lcompartments)" comment "Length axis: Calculated number of compartments"
equation "cldividers = max(0; clcompartments - 1)" comment "Length axis: Number of dividers"
equation "wcompartments = wdividers + 1" comment "Width axis: number of compartments"
equation "cwcompartments = max(0; wcompartments)" comment "Width axis: calculated number of compartments"
equation "cwdividers = max(0; cwcompartments - 1)" comment "Width axis: calculated number of dividers"
equation "d72 = hfingerw"
equation "d73 = -thickness"
equation "d75 = 2 + cwdividers"
equation "d77 = width - thickness"
equation "cwspacing = ( width - thickness ) / cwcompartments" comment "Width axis: Spacing between dividers"
equation "ldividers = 0" comment "Length axis: number of dividers"
equation "wdividers = 0" comment "Width axis: number of dividers"
equation "dividero = 40 mm" comment "Divider offset from main box"
equation "d103 = ciheight"
equation "d104 = -thickness"
equation "outerMargin = 20 mm"
equation "innerMargin = 30 mm"
equation "_sideLength = 50 mm"
equation "heightMargin = 6 mm"
equation "quantX = 3"
equation "quantY = 1"
equation "sideLength = 50 mm"
equation "outerWidth = outerMargin * 2 + quantX * sideLength"
equation "outerLength = outerMargin * 2 + quantY * sideLength"
equation "innerLength = quantY * sideLength"
equation "innerWidth = quantX * sideLength"
equation "outerHeight = sideLength + 2 * heightMargin"
equation "d118 = sideLength"
equation "d119 = sideLength * quantY"
equation "d120 = -thickness"
equation "d122 = -length"
equation "d123 = thickness"
equation "d125 = -height"
equation "d126 = thickness"
equation "d130 = -thickness"
equation "d134 = -thickness"
equation "d136 = quantX * sideLength"
equation "d137 = sideLength"
equation "d138 = -thickness"
equation "d140 = quantX * sideLength"
equation "d141 = sideLength"
equation "d142 = -thickness"
equation "d144 = cilength"
equation "d145 = ciwidth"
equation "d146 = quantY * sideLength"
equation "d147 = quantX * sideLength"
equation "d148 = thickness"
equation "d150 = quantY * sideLength"
equation "d151 = sideLength"
equation "d152 = quantY * sideLength"
equation "d153 = quantX * sideLength"
named bodies: "Bottom Panel", "Front Panel", "Back Panel", "Left Panel"
